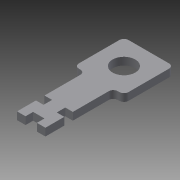
# Autodesk Inventor part: pitch_support
Saved by Autodesk Inventor 2015 (Build 190159000, 159)
## iProperties
Created: 2015-12-01
Part Number: pitch_support
Material: Generic
Document SubType Name: Modeling
Designer: jufranz
Density: 1 g/cm^3
Appearance: Default
Author: jufranz
Autodesk Inventor part; units mm, degrees
ref_plane "YZ Plane" through (0, 0, 0) normal (1, 0, 0) x (0, 1, 0)
ref_plane "XZ Plane" through (0, 0, 0) normal (0, 1, 0) x (-1, 0, 0)
ref_plane "XY Plane" through (0, 0, 0) normal (0, 0, 1) x (1, 0, 0)
sketch "Sketch1" plane through (0, 0, 0) normal (0, 1, 0) x (-1, 0, 0)
  line L0 (17.5, 14.325) -> (17.5, -14.325)
  line L1 (14.325, -17.5) -> (-14.325, -17.5)
  line L2 (-17.5, -14.325) -> (-17.5, 14.325)
  line L3 (-14.325, 17.5) -> (-13.175, 17.5)
  line L4 (-10, 20.675) -> (-10, 60)
  line L5 (-10, 60) -> (10, 60)
  line L6 (10, 60) -> (10, 20.675)
  line L7 (13.175, 17.5) -> (14.325, 17.5)
  arc A0 (10, 20.675) -> (13.175, 17.5) centre (13.175, 20.675) ccw
  arc A1 (-13.175, 17.5) -> (-10, 20.675) centre (-13.175, 20.675) ccw
  arc A2 (17.5, 14.325) -> (14.325, 17.5) centre (14.325, 14.325) ccw
  arc A3 (14.325, -17.5) -> (17.5, -14.325) centre (14.325, -14.325) ccw
  arc A4 (-17.5, -14.325) -> (-14.325, -17.5) centre (-14.325, -14.325) ccw
  arc A5 (-14.325, 17.5) -> (-17.5, 14.325) centre (-14.325, 14.325) ccw
  point P0 (0, 0)
  point P1 (17.5, 17.5)
  point P2 (17.5, -17.5)
  point P3 (-17.5, -17.5)
  point P4 (-17.5, 17.5)
  point P5 (-10, 17.5)
  point P6 (10, 17.5)
  point P7 (17.5, 0)
  point P8 (0, -17.5)
  point P9 (0, 60)
  dimension "d0" = 35
  dimension "d1" = 35
  dimension "d2" = 20
  dimension "d3" = 60
  dimension "d26" = 3.175
  dimension "d27" = 3.175
  constraints: 16 end point, 13 point on line, 12 point on circle, 12 tangent, 7 perpendicular, 6 centre point, 4 equal radius, 3 midpoint, 2 vertical alignment, 1 horizontal alignment, 1 vertical
  measures "d0" distance of point (17.5, 17.5) point (17.5, -17.5)
  measures "d1" distance of point (17.5, -17.5) point (-17.5, -17.5)
  measures "d2" distance between parallel lines of L4 L6
  measures "d3" distance from line of point (0, 0) L5
  measures "d26" radius of A0
  measures "d27" radius of A2
extrude "Extrusion1" add sketch "Sketch1" along normal blind 5.334
sketch "Sketch3" plane through (0, 5.334, 0) normal (0, 1, 0) x (1, 0, 0)
  point P0 (0, 0)
  point P1 (0, 0)
  constraints: 1 coincident
hole "Hole2" at (0, 5.334, 0) direction (0, -1, 0) diameter 16 end through all
sketch "Sketch6" plane through (10, 0, 60) normal (1, 0, 0) x (0, 0, -1)
  line L0 (0, 5.334) -> (39.325, 5.334) projected
  line L1 (0, 0) -> (39.325, 0) projected
  line L2 (14, 5.334) -> (8, 5.334)
  line L3 (8, 5.334) -> (8, 0)
  line L4 (8, 0) -> (14, 0)
  line L5 (14, 0) -> (14, 5.334)
  line L6 (0, 0) -> (0, 5.334) projected
  point P0 (60, 0)
  dimension "d41" = 6
  dimension "d42" = 8
  constraints: 8 end point, 2 parallel, 2 point on line, 1 horizontal, 1 perpendicular
  measures "d41" distance between parallel lines of L3 L5
  measures "d42" distance between parallel lines of L6 L3
extrude "Extrusion3" cut sketch "Sketch6" against normal blind 5.334 contours L0 L5 L1 L3
sketch "Sketch5" plane through (-10, 0, 60) normal (0, 0, 1) x (1, 0, 0)
  line L0 (0, 5.334) -> (20, 5.334) projected
  line L1 (0, 0) -> (6, 0)
  line L2 (6, 0) -> (6, 5.334)
  line L3 (6, 5.334) -> (0, 5.334)
  line L4 (0, 5.334) -> (0, 0)
  line L5 (20, 0) -> (14, 0)
  line L6 (14, 0) -> (14, 5.334)
  line L7 (14, 5.334) -> (20, 5.334)
  line L8 (20, 5.334) -> (20, 0)
  line L9 (20, 0) -> (20, 5.334) projected
  point P0 (10, 0)
  point P1 (20, 2.667)
  dimension "d45" = 6
  dimension "d46" = 6
  constraints: 16 end point, 4 parallel, 3 point on line, 2 horizontal, 2 midpoint, 2 perpendicular
  measures "d45" distance between parallel lines of L8 L6
  measures "d46" distance between parallel lines of L4 L2
extrude "Extrusion2" add sketch "Sketch5" along normal blind 5.334
mirror "Mirror1" about plane through (0, 0, 0) normal (1, 0, 0) of "Extrusion3"
equation "\"d46\" = d45"
body "Solid1"
